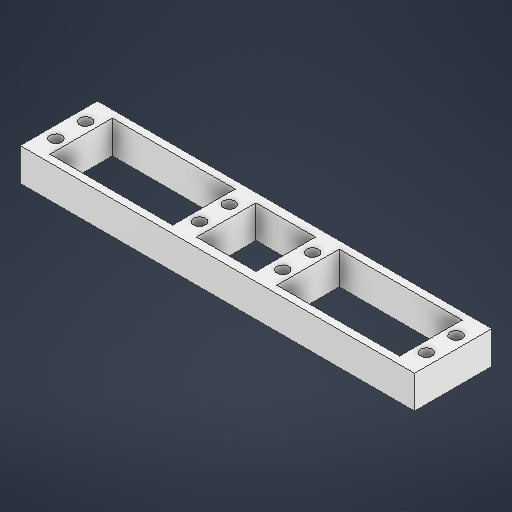
# Autodesk Inventor part: femur
Saved by Autodesk Inventor 2026.1 (Build 301233000, 233)
## iProperties
Created: 2025-08-25
Part Number: femur
Material: Generic
Document SubType Name: Modeling
Designer: emanuel
Density: 1 g/cm^3
Appearance: Default
Author: emanuel
Autodesk Inventor part; units mm, degrees
ref_plane "YZ Plane" through (0, 0, 0) normal (1, 0, 0) x (0, 1, 0)
ref_plane "XZ Plane" through (0, 0, 0) normal (0, 1, 0) x (-1, 0, 0)
ref_plane "XY Plane" through (0, 0, 0) normal (0, 0, 1) x (1, 0, 0)
sketch "Sketch1" plane through (0, 0, 0) normal (0, 1, 0) x (-1, 0, 0)
  line L0 (0, 0) -> (8, 0)
  line L1 (8, 0) -> (8, -20)
  line L2 (8, -20) -> (0, -20)
  line L3 (0, -20) -> (0, 0)
  line L4 (8, 0) -> (4, 0)
  line L5 (4, 0) -> (4, -5)
  line L6 (4, -5) -> (8, -5)
  line L7 (8, -5) -> (8, 0)
  line L8 (8, -20) -> (4, -20)
  line L9 (4, -20) -> (4, -15)
  line L10 (4, -15) -> (8, -15)
  line L11 (8, -15) -> (8, -20)
  circle A0 centre (4, -5) radius 2
  circle A1 centre (4, -15) radius 2
  line L12 (8, 0) -> (48.3, 0)
  line L13 (48.3, 0) -> (48.3, -20)
  line L14 (48.3, -20) -> (8, -20)
  line L15 (8, -20) -> (8, 0)
  line L16 (48.3, 0) -> (56.3, 0)
  line L17 (56.3, 0) -> (56.3, -20)
  line L18 (56.3, -20) -> (48.3, -20)
  line L19 (48.3, -20) -> (48.3, 0)
  line L20 (56.3, 0) -> (52.3, 0)
  line L21 (52.3, 0) -> (52.3, -5)
  line L22 (52.3, -5) -> (56.3, -5)
  line L23 (56.3, -5) -> (56.3, 0)
  line L24 (56.3, -20) -> (52.3, -20)
  line L25 (52.3, -20) -> (52.3, -15)
  line L26 (52.3, -15) -> (56.3, -15)
  line L27 (56.3, -15) -> (56.3, -20)
  circle A2 centre (52.3, -5) radius 2
  circle A3 centre (52.3, -15) radius 2
  line L28 (56.3, -20) -> (0, -20)
  line L29 (0, -20) -> (0, -23)
  line L30 (0, -23) -> (56.3, -23)
  line L31 (56.3, -23) -> (56.3, -20)
  line L32 (56.3, 0) -> (0, 0)
  line L33 (0, 0) -> (0, 3)
  line L34 (0, 3) -> (56.3, 3)
  line L35 (56.3, 3) -> (56.3, 0)
  line L36 (0, -23) -> (-20, -23)
  line L37 (-20, -23) -> (-20, 3)
  line L38 (0, 3) -> (0, -23)
  line L39 (0, -20) -> (-20, -20)
  line L40 (-20, -20) -> (-20, 0)
  line L41 (-20, 0) -> (0, 0)
  line L42 (0, 0) -> (0, -20)
  line L43 (-20, -20) -> (-28, -20)
  line L44 (-28, -20) -> (-28, 0)
  line L45 (-28, 0) -> (-20, 0)
  line L46 (-20, 0) -> (-20, -20)
  line L47 (-28, -20) -> (-68.3, -20)
  line L48 (-68.3, -20) -> (-68.3, 0)
  line L49 (-68.3, 0) -> (-28, 0)
  line L50 (-28, 0) -> (-28, -20)
  line L51 (-68.3, -20) -> (-76.3, -20)
  line L52 (-76.3, -20) -> (-76.3, 0)
  line L53 (-76.3, 0) -> (-68.3, 0)
  line L54 (-68.3, 0) -> (-68.3, -20)
  line L55 (-20, -20) -> (-76.3, -20)
  line L56 (-76.3, -20) -> (-76.3, -23)
  line L57 (-76.3, -23) -> (-20, -23)
  line L58 (-20, -23) -> (-20, -20)
  line L59 (-20, 0) -> (-76.3, 0)
  line L60 (-76.3, 0) -> (-76.3, 3)
  line L61 (-76.3, 3) -> (-20, 3)
  line L62 (-20, 3) -> (-20, 0)
  line L63 (-20, -20) -> (-24, -20)
  line L64 (-24, -20) -> (-24, -15)
  line L65 (-24, -15) -> (-20, -15)
  line L66 (-20, -15) -> (-20, -20)
  line L67 (-20, 0) -> (-24, 0)
  line L68 (-24, 0) -> (-24, -5)
  line L69 (-24, -5) -> (-20, -5)
  line L70 (-20, -5) -> (-20, 0)
  line L71 (-76.3, -20) -> (-72.3, -20)
  line L72 (-72.3, -20) -> (-72.3, -15)
  line L73 (-72.3, -15) -> (-76.3, -15)
  line L74 (-76.3, -15) -> (-76.3, -20)
  line L75 (-76.3, 0) -> (-72.3, 0)
  line L76 (-72.3, 0) -> (-72.3, -5)
  line L77 (-72.3, -5) -> (-76.3, -5)
  line L78 (-76.3, -5) -> (-76.3, 0)
  circle A4 centre (-24, -15) radius 2
  circle A5 centre (-24, -5) radius 2
  circle A6 centre (-72.3, -15) radius 2
  circle A7 centre (-72.3, -5) radius 2
  line L79 (0, 3) -> (-20, 3)
  point P0 (0, 0)
  point P1 (-28, 0)
  point P2 (-20, 3)
  point P3 (-20, 3)
  point P4 (8, -20)
  point P5 (-20, 3)
  dimension "d0" = 8
  dimension "d1" = 20
  dimension "d2" = 4
  dimension "d3" = 5
  dimension "d4" = 4
  dimension "d5" = 5
  dimension "d6" = 4
  dimension "d7" = 4
  dimension "d8" = 40.3
  dimension "d9" = 8
  dimension "d10" = 4
  dimension "d11" = 5
  dimension "d12" = 4
  dimension "d13" = 5
  dimension "d14" = 4
  dimension "d15" = 4
  dimension "d16" = 3
  dimension "d17" = 3
  dimension "d18" = 20
  dimension "d19" = 8
  dimension "d20" = 40.3
  dimension "d21" = 8
  dimension "d22" = 4
  dimension "d23" = 5
  dimension "d24" = 4
  dimension "d25" = 5
  dimension "d26" = 4
  dimension "d27" = 5
  dimension "d28" = 4
  dimension "d29" = 5
  dimension "d30" = 4
  dimension "d31" = 4
  dimension "d32" = 4
  dimension "d33" = 4
  dimension "d36" = 3
  dimension "d37" = 3
  constraints: 160 end point, 39 parallel, 20 horizontal, 20 perpendicular, 8 centre point, 8 coincident, 5 point on line, 1 collinear
  measures "d0" distance of L1.end L2.end
  measures "d1" distance of L0.end L1.end
  measures "d2" distance of L6.end L5.end
  measures "d3" distance of L5.end L4.end
  measures "d4" distance of L9.end L10.end
  measures "d5" distance of L8.end L9.end
  measures "d6" diameter of A0
  measures "d7" diameter of A1
  measures "d8" distance of L13.end L14.end
  measures "d9" distance of L17.end L18.end
  measures "d10" distance of L22.end L21.end
  measures "d11" distance of L21.end L20.end
  measures "d12" distance of L25.end L26.end
  measures "d13" distance of L24.end L25.end
  measures "d14" diameter of A2
  measures "d15" diameter of A3
  measures "d16" distance of L29.end L28.end
  measures "d17" distance of L32.end L33.end
  measures "d18" distance of L37.end L38.start
  measures "d19" distance of L44.end L45.end
  measures "d20" distance of L48.end L49.end
  measures "d21" distance of L52.end L53.end
  measures "d22" distance of L64.end L65.end
  measures "d23" distance of L63.end L64.end
  measures "d24" distance of L69.end L68.end
  measures "d25" distance of L68.end L67.end
  measures "d26" distance of L73.end L72.end
  measures "d27" distance of L72.end L71.end
  measures "d28" distance of L76.end L77.end
  measures "d29" distance of L75.end L76.end
  measures "d30" diameter of A4
  measures "d31" diameter of A5
  measures "d32" diameter of A6
  measures "d33" diameter of A7
  measures "d36" distance between parallel lines of L47 L57
  measures "d37" distance between parallel lines of L49 L61
extrude "Extrusion1" add sketch "Sketch1" along normal blind 11 contours L33 L34 L35 L16 L12 L0 | L0 L5 A0 L6 L1 L10 A1 L9 L2 L3 | L41 L37 L79 L33 | L0 L1 L6 A0 L5 | L2 L14 L18 L31 L30 L29 | L29 L36 L37 L39 | L45 L49 L53 L60 L61 L37 | L37 L69 A5 L68 L45 | L9 A1 L10 L1 L2 | L43 L64 A4 L65 L37 | L37 L57 L56 L51 L47 L43 | L37 L65 A4 L64 L43 L44 L45 L68 A5 L69 | L16 L21 A2 L22 L17 L26 A3 L25 L18 L13 | L17 L22 A2 L21 L16 | L18 L25 A3 L26 L17 | L53 L76 A7 L77 L52 | L48 L51 L72 A6 L73 L52 L77 A7 L76 L53 | L52 L73 A6 L72 L51
sketch "Sketch2" plane through (0, 11, 0) normal (0, 1, 0) x (1, 0, 0)
  line L0 (-48.3, 0) -> (-48.3, 20) projected
  line L1 (-48.3, 20) -> (-48.8, 20)
  line L2 (-48.8, 20) -> (-48.8, 20.5)
  line L3 (-48.8, 20.5) -> (-48.3, 20.5)
  line L4 (-48.3, 20.5) -> (-48.3, 20)
  line L5 (-48.8, 20.5) -> (-7.5, 20.5)
  line L6 (-7.5, 20.5) -> (-7.5, -0.5)
  line L7 (-7.5, -0.5) -> (-48.8, -0.5)
  line L8 (-48.8, -0.5) -> (-48.8, 20.5)
  line L9 (28, 0) -> (28, 20) projected
  line L10 (28, 20) -> (27.5, 20)
  line L11 (27.5, 20) -> (27.5, 20.5)
  line L12 (27.5, 20.5) -> (28, 20.5)
  line L13 (28, 20.5) -> (28, 20)
  line L14 (27.5, 20.5) -> (68.8, 20.5)
  line L15 (68.8, 20.5) -> (68.8, -0.5)
  line L16 (68.8, -0.5) -> (27.5, -0.5)
  line L17 (27.5, -0.5) -> (27.5, 20.5)
  point P0 (0, 0)
  dimension "d39" = 0.5
  dimension "d40" = 0.5
  dimension "d41" = 41.3
  dimension "d42" = 21
  dimension "d43" = 0.5
  dimension "d44" = 0.5
  dimension "d45" = 41.3
  dimension "d46" = 21
  constraints: 32 end point, 8 parallel, 4 horizontal, 4 perpendicular
  measures "d39" distance of L2.end L3.end
  measures "d40" distance of L1.end L2.end
  measures "d41" distance of L6.end L7.end
  measures "d42" distance of L5.end L6.end
  measures "d43" distance of L11.end L12.end
  measures "d44" distance of L10.end L11.end
  measures "d45" distance of L15.end L16.end
  measures "d46" distance of L14.end L15.end
extrude "Extrusion2" cut sketch "Sketch2" against normal blind 11
body "Solid1"
